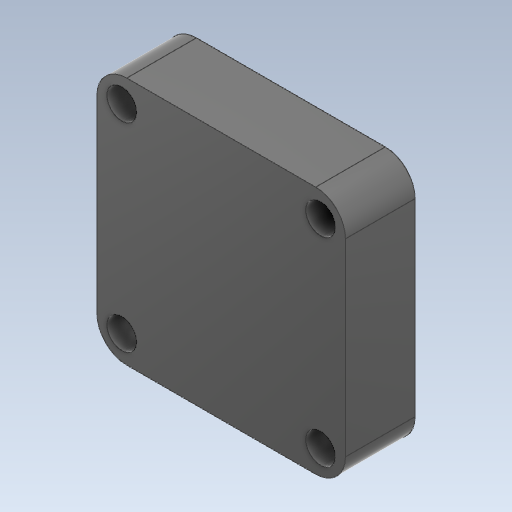
# Autodesk Inventor part: YDM2507C12F
Saved by Autodesk Inventor 2020 (Build 240168000, 168)
## iProperties
Part Number: YDM2507C12F
Material: 一般
Document SubType Name: Modeling
Designer: Masato Kubotera
Density: 1 g/cm^3
Appearance: 滑らか - 黒
Catalog Web Link: https://akizukidenshi.com/catalog/g/gP-16826/
Description: ReadyMade
Author: Masato Kubotera
Autodesk Inventor part; units mm, degrees
ref_plane "YZ Plane" through (0, 0, 0) normal (1, 0, 0) x (0, 1, 0)
ref_plane "XZ Plane" through (0, 0, 0) normal (0, 1, 0) x (-1, 0, 0)
ref_plane "XY Plane" through (0, 0, 0) normal (0, 0, 1) x (1, 0, 0)
sketch "スケッチ1" plane through (0, 0, 0) normal (0, 0, 1) x (1, 0, 0)
  line L0 (-12.5, 12.5) -> (12.5, 12.5)
  line L1 (12.5, 12.5) -> (12.5, -12.5)
  line L2 (12.5, -12.5) -> (-12.5, -12.5)
  line L3 (-12.5, -12.5) -> (-12.5, 12.5)
  line L4 (-12.5, 12.5) -> (12.5, -12.5) construction
  line L5 (12.5, 12.5) -> (-12.5, -12.5) construction
  line L6 (10, 10) -> (-10, 10) construction
  line L7 (-10, 10) -> (-10, -10) construction
  line L8 (-10, -10) -> (10, -10) construction
  line L9 (10, -10) -> (10, 10) construction
  line L10 (10, 10) -> (-10, -10) construction
  line L11 (-10, 10) -> (10, -10) construction
  circle A0 centre (-10, 10) radius 1.5
  circle A1 centre (10, 10) radius 1.5
  circle A2 centre (-10, -10) radius 1.5
  circle A3 centre (10, -10) radius 1.5
  point P0 (0, 0)
  dimension "d0" = 25
  dimension "d1" = 25
  dimension "d2" = 20
  dimension "d3" = 20
  dimension "d4" = 3
  dimension "d5" = 3
  dimension "d6" = 3
  dimension "d7" = 3
  constraints: 24 end point, 4 centre point, 4 coincident, 4 midpoint, 4 parallel, 2 horizontal, 2 perpendicular
  measures "d0" distance of L1.end L2.end
  measures "d1" distance of L0.end L1.end
  measures "d2" distance of L8.end L7.end
  measures "d3" distance of L7.end L6.end
  measures "d4" diameter of A0
  measures "d5" diameter of A1
  measures "d6" diameter of A2
  measures "d7" diameter of A3
extrude "押し出し1" add sketch "スケッチ1" along normal blind 7
fillet "フィレット1" radius 3 4 edges at (-12.5, 12.5, 3.5) (12.5, 12.5, 3.5) (12.5, -12.5, 3.5) (-12.5, -12.5, 3.5)
